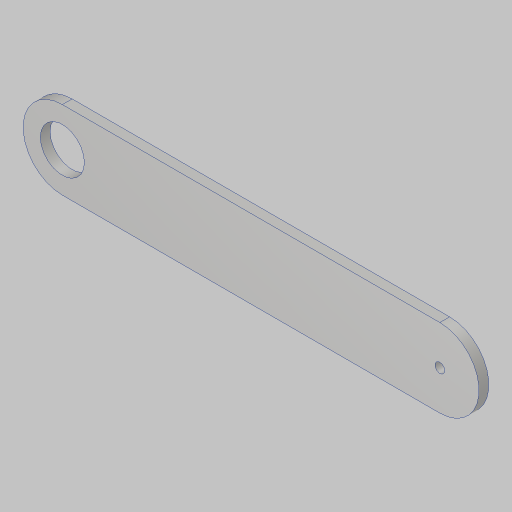
# Autodesk Inventor part: GP4-004
Saved by Autodesk Inventor 2023.5 (Build 275446000, 446)
## iProperties
Created: 2025-02-23
Part Number: GP4-004
Material: Aluminum 6061
Document SubType Name: Modeling
Designer: slick
Density: 2.7 g/cm^3
Appearance: Aluminum - Flat
Author: slick
Autodesk Inventor part; units mm, degrees
ref_plane "YZ Plane" through (0, 0, 0) normal (1, 0, 0) x (0, 1, 0)
ref_plane "XZ Plane" through (0, 0, 0) normal (0, 1, 0) x (-1, 0, 0)
ref_plane "XY Plane" through (0, 0, 0) normal (0, 0, 1) x (1, 0, 0)
sketch "Sketch1" plane through (0, 0, 0) normal (0, 0, 1) x (1, 0, 0)
  circle A0 centre (0, 0) radius 14.2875
  circle A1 centre (244.475, 0) radius 3.175
  line L0 (0, 0) -> (244.475, 0) construction
  line L1 (0, 0) -> (244.475, 0) construction
  line L2 (0, -25.4) -> (244.475, -25.4)
  line L3 (244.475, 25.4) -> (0, 25.4)
  arc A2 (0, 25.4) -> (0, -25.4) centre (0, 0) ccw
  arc A3 (244.475, -25.4) -> (244.475, 25.4) centre (244.475, 0) ccw
  point P0 (122.2375, 0)
  dimension "d0" = 28.575
  dimension "d1" = 244.475
  dimension "d2" = 50.8
  dimension "d3" = 6.35
  constraints: 10 end point, 4 centre point, 4 point on circle, 4 tangent, 2 equal length, 1 coincident, 1 horizontal, 1 midpoint
  measures "d0" diameter of A0
  measures "d1" distance of L0.start L0.end
  measures "d2" diameter of A3
  measures "d3" diameter of A1
extrude "Extrusion1" add sketch "Sketch1" along normal blind 6.35
body "Solid1"
